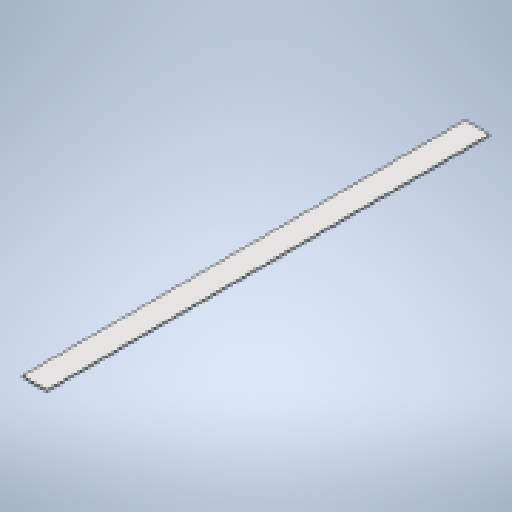
# Autodesk Inventor part: BSH 504 inner cross
Saved by Autodesk Inventor 2025 (Build 290162010, 162A)
## iProperties
Created: 2024-09-03
Part Number: BSH 504 inner cross
Material: Stainless Steel
Document SubType Name: Sheet Metal
Designer: pokla
Density: 8 g/cm^3
Sheet Metal Rule: AISI304 3mm Die 32
Sheet Metal Width: 0,000 mm
Sheet Metal Length: 0,000 mm
Sheet Metal Area: 0,000 mm^2
Appearance: Default
Author: pokla
Autodesk Inventor part; units mm, degrees
ref_plane "YZ Plane" through (0, 0, 0) normal (1, 0, 0) x (0, 1, 0)
ref_plane "XZ Plane" through (0, 0, 0) normal (0, 1, 0) x (-1, 0, 0)
ref_plane "XY Plane" through (0, 0, 0) normal (0, 0, 1) x (1, 0, 0)
sketch "Sketch1" plane through (0, 0, 0) normal (0, 0, 1) x (1, 0, 0)
  circle A0 centre (0, 0) radius 550 construction
  circle A1 centre (0, 0) radius 450
  line L0 (0, 450) -> (0, -450) construction
  line L1 (450, 0) -> (-450, 0)
  line L2 (25, 449.305) -> (25, -449.305)
  line L3 (-25, 449.305) -> (-25, -449.305)
  point P0 (0, 0)
  point P1 (-25, 0)
  point P2 (25, 0)
  dimension "d12" = 900
  dimension "d11" = 1100
  dimension "d13" = 25
  dimension "d14" = 25
  measures "d11" diameter of A0
  measures "d13" distance between parallel lines of L0 L2
  measures "d14" distance between parallel lines of L0 L3
extrude "Plate2" add sketch "Sketch1" against normal blind 3 contours A1 L3 L1 L2 picked at (2.779, -149.9743)
equation "\"d12\" = d11 - 2 * Ширина_кольца"
equation "\"d11\" = Диаметр_вн"
equation "\"d13\" = 0.5 * Ширина_креста"
equation "\"d14\" = d13"
equation "\"d15\" = Thickness"
equation "\"BendReliefWidth\" = Thickness"
equation "\"BendReliefDepth\" = 0.5 * Thickness"
equation "\"CornerReliefSize\" = 4 * Thickness"
equation "\"MinimumRemnant\" = 2 * Thickness"
equation "\"TransitionRadius\" = BendRadius"
equation "\"JacobiRadiusSize\" = BendRadius"
equation "\"GapSize\" = Thickness"
equation "\"Ширина_кольца\" = 100"
equation "\"Диаметр_вн\" = 1100"
equation "\"Ширина_креста\" = 50"
equation "\"Thickness\" = 3"
equation "\"BendRadius\" = 5"
body "Solid2"
